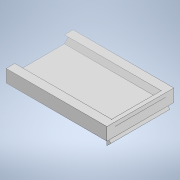
# Autodesk Inventor part: Enclosure-Bottom
Saved by Autodesk Inventor 2020 (Build 240168000, 168)
## iProperties
Created: 2019-07-15
Part Number: Enclosure-Bottom
Material: Generic
Document SubType Name: Modeling
Designer: tyrre
Density: 1 g/cm^3
Appearance: Default
Author: tyrre
Autodesk Inventor part; units mm, degrees
ref_plane "YZ Plane" through (0, 0, 0) normal (1, 0, 0) x (0, 1, 0)
ref_plane "XZ Plane" through (0, 0, 0) normal (0, 1, 0) x (-1, 0, 0)
ref_plane "XY Plane" through (0, 0, 0) normal (0, 0, 1) x (1, 0, 0)
sketch "Sketch5" plane through (0, 0, 0) normal (0, 0, 1) x (1, 0, 0)
  line L0 (-32, -5) -> (32, -5)
  line L1 (32, -5) -> (32, 5)
  line L2 (32, 5) -> (-32, 5)
  line L3 (-32, 5) -> (-32, -5)
  line L4 (-32, -5) -> (32, 5) construction
  line L5 (32, -5) -> (-32, 5) construction
  point P0 (0, 0)
  dimension "d17" = 64
  dimension "d18" = 10
  constraints: 12 end point, 2 midpoint, 2 parallel, 1 horizontal, 1 perpendicular
  measures "d17" distance of L2.end L1.end
  measures "d18" distance of L1.end L0.end
extrude "Extrusion5" add sketch "Sketch5" along normal mid plane 46.5
ref_plane "Work Plane2" through (0, 0, 15.75) normal (0, 0, 1) x (1, 0, 0)
sketch "Sketch7" plane through (0, 0, 15.75) normal (0, 0, 1) x (1, 0, 0)
  line L0 (32, 5) -> (-32, 5) projected
  line L1 (-32, 5) -> (-32, -5) projected
  line L2 (-32, -5) -> (32, -5) projected
  line L3 (32, -5) -> (32, 5) projected
  line L4 (32, -5) -> (32, 5) projected
  line L5 (-32, -5) -> (32, -5) projected
  line L6 (32, 5) -> (-32, 5) projected
  line L7 (29.5, 5) -> (29.5, 0)
  line L8 (29.5, 5) -> (32, 2.5)
  line L9 (32, 2.5) -> (29.5, 0)
  point P0 (0, 0)
  constraints: 6 end point, 1 point on line
extrude "Extrusion6" cut sketch "Sketch7" against normal blind 31.5 contours L8 L9 L7
sketch "Sketch8" plane through (-32, -5, 23.25) normal (-1, 0, 0) x (0, 0, 1)
  line L0 (-46.5, 10) -> (0, 10) projected
  line L1 (-46.5, 10) -> (-41.5, 10)
  line L2 (-41.5, 0) -> (-46.5, 0)
  line L3 (-46.5, 5) -> (-46.5, 10)
  line L4 (0, 10) -> (-5, 10)
  line L5 (-46.5, 0) -> (-46.5, 10) projected
  line L6 (-41.5, 10) -> (-39, 10)
  line L7 (-39, 10) -> (-41.5, 7.5)
  line L8 (-39, 7.5) -> (-39, 5) projected
  line L9 (-39, 5) -> (-41.5, 7.5)
  line L10 (-5, 10) -> (-7.5, 10)
  line L11 (-7.5, 10) -> (-5, 7.5)
  line L12 (-7.5, 5) -> (-7.5, 7.5) projected
  line L13 (-5, 7.5) -> (-7.5, 5)
  line L14 (-7.5, 5) -> (-39, 5)
  line L15 (-39, 10) -> (-39, 7.5) projected
  line L16 (-7.5, 7.5) -> (-7.5, 10) projected
  line L17 (-39, 10) -> (-7.5, 10)
  line L18 (-39, 10) -> (-7.5, 10)
  line L19 (-7.5, 5) -> (-39, 5) projected
  line L20 (-39, 5) -> (-7.5, 5)
  point P0 (-23.25, 5)
  constraints: 28 end point, 4 point on line, 3 perpendicular, 2 equal length, 1 horizontal, 1 midpoint
extrude "Extrusion8" cut sketch "Sketch8" against normal blind 61.5
sketch "Sketch9" plane through (-32, -5, -23.25) normal (-1, 0, 0) x (0, 0, 1)
  line L0 (0, 10) -> (46.5, 10) projected
  line L1 (0, 10) -> (2, 10)
  line L2 (2, 10) -> (2, 0)
  line L3 (2, 0) -> (0, 0)
  line L4 (0, 0) -> (0, 10)
  line L5 (46.5, 10) -> (44.5, 10)
  line L6 (44.5, 10) -> (44.5, 0)
  line L7 (44.5, 0) -> (46.5, 0)
  line L8 (46.5, 0) -> (46.5, 10)
  point P0 (23.25, 5)
  dimension "d37" = 2
  dimension "d38" = 2
  constraints: 16 end point, 4 parallel, 3 point on line, 2 perpendicular
  measures "d37" distance of L0.start L1.end
  measures "d38" distance of L5.start L5.end
extrude "Extrusion9" cut sketch "Sketch9" against normal through all
sketch "Sketch10" plane through (-32, 0, -15.75) normal (-1, 0, 0) x (0, 0, 1)
  line L0 (-5.5, -5) -> (-5.5, 5) projected
  line L1 (37, 5) -> (37, -5) projected
  line L2 (-5.5, -5) -> (37, -5)
  line L3 (37, -5) -> (37, -8)
  line L4 (37, -8) -> (-5.5, -8)
  line L5 (-5.5, -8) -> (-5.5, -5)
  point P0 (15.75, 0)
  dimension "d70" = 3
  constraints: 8 end point, 2 parallel, 1 horizontal, 1 perpendicular
  measures "d70" distance of L1.end L3.end
sketch "Sketch12" plane through (-32, 0, -15.75) normal (-1, 0, 0) x (0, 0, 1)
  line L0 (37, -3) -> (42, -3)
  line L1 (42, -3) -> (42, 5)
  line L2 (42, 5) -> (37, 5)
  line L3 (37, 5) -> (37, -3)
  point P0 (15.75, 0)
  dimension "d56" = 5
  dimension "d59" = 8
  constraints: 8 end point, 2 parallel, 1 horizontal, 1 perpendicular
  measures "d56" distance of L2.end L1.end
  measures "d59" distance of L0.end L1.end
revolve "Revolution1" [suppressed]
sketch "Sketch13" plane through (-32, -3, 21.25) normal (-1, 0, 0) x (0, 0, 1)
  line L0 (5, 8) -> (0, 8) projected
  line L1 (0, 8) -> (0, 0) projected
  line L2 (0, 0) -> (5, 0) projected
  line L3 (5, 0) -> (5, 8) projected
  line L4 (5, 0) -> (5, 8) projected
  line L5 (5, 4) -> (4, 4)
  point P0 (-21.25, 3)
  dimension "d58" = 1
  constraints: 2 end point, 1 coincident, 1 horizontal, 1 midpoint
  measures "d58" distance of L5.start L5.end
feature "Snap Fit2" [suppressed]
mirror "Mirror1" [suppressed]
extrude "Extrusion11" add sketch "Sketch10" against normal blind 64
sketch "Sketch14" plane through (-32, 0, -15.75) normal (-1, 0, 0) x (0, 0, 1)
  line L0 (37, -8) -> (37, 5) projected
  line L1 (31.5, 5) -> (37, 5) projected
  line L2 (31.5, 5) -> (34, 2.5) projected
  line L3 (34, 2.5) -> (31.5, 0) projected
  line L4 (31.5, 0) -> (0, 0) projected
  line L5 (0, 0) -> (-2.5, 2.5) projected
  line L6 (-2.5, 2.5) -> (0, 5) projected
  line L7 (-5.5, 5) -> (0, 5) projected
  line L8 (-5.5, 5) -> (-5.5, -8) projected
  line L9 (-5.5, -8) -> (37, -8) projected
  line L10 (-5.5, -8) -> (37, -8) projected
  line L11 (0, -3) -> (-2.5, -5.5)
  line L12 (0, -8) -> (-2.5, -5.5)
  line L13 (0, -8) -> (-5.5, -8)
  line L14 (-5.5, 5) -> (-5.5, -8) projected
  line L15 (-5.5, 0) -> (-5, 0)
  line L16 (-5.5, -3) -> (-5.5, -8)
  line L17 (31.5, -3) -> (34, -5.5)
  line L18 (31.5, -8) -> (34, -5.5)
  line L19 (31.5, -8) -> (37, -8)
  line L20 (37, -3) -> (37, -8)
  line L21 (0, -3) -> (-5.5, -3)
  line L22 (31.5, -3) -> (37, -3)
  line L23 (37, -8) -> (37, 5) projected
  point P0 (15.75, 0)
  constraints: 22 end point, 4 point on line, 3 perpendicular, 2 collinear
extrude "Extrusion12" cut sketch "Sketch14" against normal blind 61.5 contours L9 L18 L17 L22 L0 | L9 L8 L21 L11 L12
sketch "Sketch15" plane through (32, 5, 21.25) normal (1, 0, 0) x (0, 0, -1)
  line L0 (0, -13) -> (42.5, -13) projected
  line L1 (0, -13) -> (2.5, -13)
  line L2 (2.5, -13) -> (2.5, -8)
  line L3 (2.5, -8) -> (0, -8)
  line L4 (0, -8) -> (0, -13)
  line L5 (42.5, -13) -> (42.5, -8) projected
  line L6 (42.5, -13) -> (40, -13)
  line L7 (40, -13) -> (40, -8)
  line L8 (40, -8) -> (42.5, -8)
  line L9 (42.5, -8) -> (42.5, -13)
  point P0 (21.25, -5)
  dimension "d76" = 2.5
  dimension "d77" = 5
  dimension "d78" = 2.5
  dimension "d79" = 5
  constraints: 16 end point, 4 parallel, 2 perpendicular, 2 point on line
  measures "d76" distance of L0.start L1.end
  measures "d77" distance of L2.end L1.end
  measures "d78" distance of L0.end L6.end
  measures "d79" distance of L6.end L7.end
extrude "Extrusion13" cut sketch "Sketch15" against normal blind 2.5
sketch "Sketch16" plane through (32, -8, 18.75) normal (0, 0, 1) x (1, 0, 0)
  line L0 (-2.5, 5) -> (-2.5, 2.5) projected
  line L1 (-2.5, 5) -> (0, 2.5)
  line L2 (0, 0) -> (0, 5) projected
  line L3 (-64, 0) -> (-2.5, 0) projected
  line L4 (-2.5, 0) -> (0, 2.5)
  line L5 (0, 5) -> (-64, 5) projected
  line L6 (-2.5, 5) -> (0, 5)
  line L7 (0, 5) -> (0, 0)
  line L8 (0, 0) -> (-2.5, 0)
  point P0 (-32, 8)
  constraints: 10 end point, 3 perpendicular, 1 collinear, 1 midpoint
extrude "Extrusion14" cut sketch "Sketch16" against normal through all
body "Solid2"
body "Solid3"
